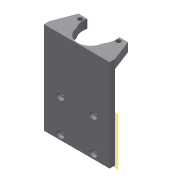
# Autodesk Inventor part: 01_WG_writer_BASE
Saved by Autodesk Inventor 2019.4 (Build 234330000, 330)
## iProperties
Created: 2020-11-13
Part Number: 01_WG_writer_BASE
Material: Generic
Document SubType Name: Modeling
Designer: diederichbenedict
Density: 1 g/cm^3
Appearance: Default
Author: diederichbenedict
Autodesk Inventor part; units mm, degrees
ref_plane "YZ Plane" through (0, 0, 0) normal (1, 0, 0) x (0, 1, 0)
ref_plane "XZ Plane" through (0, 0, 0) normal (0, 1, 0) x (-1, 0, 0)
ref_plane "XY Plane" through (0, 0, 0) normal (0, 0, 1) x (1, 0, 0)
ref_plane "Work Plane1" through (0, 0, 0) normal (0, 0, 1) x (1, 0, 0)
sketch "Sketch1" plane through (0, 0, 0) normal (0, 0, 1) x (1, 0, 0)
  circle A0 centre (-15, -15) radius 1.5 projected
  circle A1 centre (15, 15) radius 1.5 projected
  circle A2 centre (15, -15) radius 1.5 projected
  circle A3 centre (-15, 15) radius 1.5 projected
  line L0 (30, 20) -> (-30, 20) projected
  line L1 (-30, 20) -> (-30, -20) projected
  line L2 (-30, -20) -> (30, -20) projected
  line L3 (30, -20) -> (30, 20) projected
  line L4 (30, 20) -> (-30, 20)
  line L5 (-30, 20) -> (-30, 64.25)
  line L6 (-30, 64.25) -> (30, 64.25)
  line L7 (30, 64.25) -> (30, 20)
  line L8 (13.5554, 64.25) -> (17.5, 64.25) projected
  point P0 (0, 0)
  constraints: 8 end point, 2 parallel, 1 horizontal, 1 perpendicular, 1 point on line
extrude "Extrusion1" add sketch "Sketch1" along normal blind 5 contours A0 | A1 | A2 | A3 | L3 L2 L1 L0 | L0 L5 L6 L7
sketch "Sketch2" plane through (0, 0, 5) normal (0, 0, 1) x (1, 0, 0)
  circle A0 centre (15, 15) radius 1.5 projected
  circle A1 centre (15, -15) radius 1.5 projected
  circle A2 centre (-20, 13) radius 1.5 projected
  circle A3 centre (-20, -13) radius 1.5 projected
  circle A4 centre (-15, -15) radius 1.5 projected
  circle A5 centre (-15, 15) radius 1.5 projected
  point P0 (0, 0)
hole "Hole1" at (15, 15, 5) at (15, -15, 5) at (-15, -15, 5) at (-15, 15, 5) direction (0, 0, -1) diameter 3.5 depth 8 tip angle 118 counterbore diameter 7 counterbore depth 3
sketch "Sketch3" plane through (-30, 64.25, 0) normal (0, 1, 0) x (1, 0, 0)
  circle A0 centre (12.5, 15.7367) radius 2.1 projected
  circle A1 centre (47.5, 15.7367) radius 2.1 projected
  arc A2 (16, 15.7367) -> (44, 15.7367) centre (30, 15.7367) ccw projected
  circle A3 centre (30, 15.7367) radius 15
  line L0 (12.5, 19.2367) -> (16.4446, 19.2367) projected
  line L1 (43.5554, 19.2367) -> (47.5, 19.2367) projected
  line L2 (15.414, 19.2367) -> (7.414, 19.2367)
  line L3 (0, 0) -> (60, 0) projected
  line L4 (7.414, 19.2367) -> (0, 0)
  line L5 (0, 0) -> (60, 0)
  line L6 (44.586, 19.2367) -> (52.586, 19.2367)
  line L7 (52.586, 19.2367) -> (60, 0)
  circle A4 centre (12.5, 15.7367) radius 1.45
  circle A5 centre (47.5, 15.7367) radius 1.45
  point P0 (30, 0)
  dimension "d9" = 30
  dimension "d10" = 8
  dimension "d11" = 8
  dimension "d12" = 2.9
  dimension "d13" = 2.9
  constraints: 10 end point, 4 point on line, 3 centre point, 3 coincident, 2 point on circle, 1 parallel
  measures "d9" diameter of A3
  measures "d10" distance of L2.start L2.end
  measures "d11" distance of L6.start L6.end
  measures "d12" diameter of A4
  measures "d13" diameter of A5
extrude "Extrusion2" add sketch "Sketch3" against normal blind 8 contours A3 L1 L6 L7 L3 L4 L2 L0
sketch "Sketch4" plane through (-30, 64.25, 5) normal (0, 1, 0) x (1, 0, 0)
  circle A0 centre (30, 12.7367) radius 10 projected
  circle A1 centre (30, 12.7367) radius 12
  point P0 (30, 5)
  dimension "d16" = 24
  constraints: 1 centre point, 1 coincident
  measures "d16" diameter of A1
extrude "Extrusion3" cut sketch "Sketch4" against normal blind 25 contours A0 | A1
body "Solid1"
